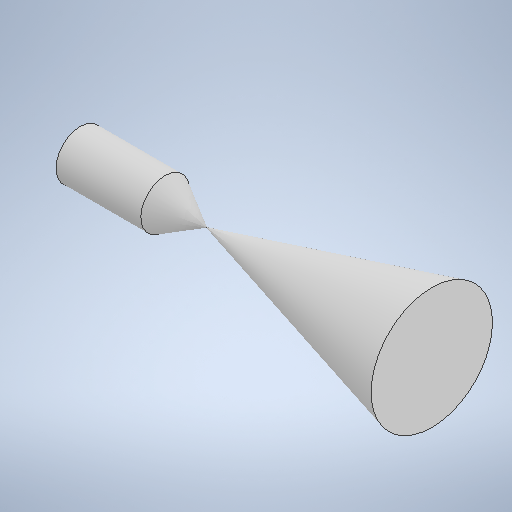
# Autodesk Inventor part: NozzlePath
Saved by Autodesk Inventor 2025.2 (Build 292293000, 293)
## iProperties
Created: 2026-05-12
Part Number: NozzlePath
Material: Generic
Document SubType Name: Modeling
Designer: Simon
Density: 1 g/cm^3
Appearance: Default
Author: Simon
Autodesk Inventor part; units mm, degrees
ref_plane "YZ Plane" through (0, 0, 0) normal (1, 0, 0) x (0, 1, 0)
ref_plane "XZ Plane" through (0, 0, 0) normal (0, 1, 0) x (-1, 0, 0)
ref_plane "XY Plane" through (0, 0, 0) normal (0, 0, 1) x (1, 0, 0)
sketch "Sketch1" plane through (0, 0, 0) normal (0, 0, 1) x (1, 0, 0)
  line L0 (0, -0.0234) -> (0, 1.9766)
  line L1 (0, 1.9766) -> (50, 1.9766)
  line L2 (0, -0.0234) -> (0, 0)
  line L3 (0, 0) -> (50, 0)
  line L4 (0, -0.0234) -> (0, 4.9766)
  line L5 (0, 4.9766) -> (50, 4.9766)
  line L6 (0, -0.0234) -> (0, 3.9766)
  line L7 (0, 3.9766) -> (4, 3.9766)
  line L8 (4, 3.9766) -> (4, 1.9766)
  line L9 (4, 1.9766) -> (4, 9.9766)
  line L10 (4, 1.9766) -> (6.7109, 1.9766) construction
  line L11 (4, 9.9766) -> (7, 9.9766)
  line L12 (7, 9.9766) -> (7, 1.9766)
  line L13 (7, 1.9766) -> (10.4235, 0)
  line L14 (7, 1.9766) -> (9.25, 1.9766) construction
  line L15 (10.4235, 0) -> (28.9964, 4.9766)
  line L16 (10.4235, 0) -> (29.6515, 0) construction
  line L17 (28.9964, 4.9766) -> (28.9964, 6.9766)
  line L18 (28.9964, 6.9766) -> (7, 9.9766)
  line L19 (0, -0.0234) -> (50, -0.0234)
  line L20 (-10, -0.0234) -> (60, -0.0234)
  line L21 (28.9964, 4.9766) -> (28.9964, -0.0234)
  point P0 (28.9964, -0.0234)
  dimension "d0" = 2
  dimension "d1" = 50
  dimension "d2" = 0.0234
  dimension "d3" = 5
  dimension "d4" = 4
  dimension "d5" = 4
  dimension "d6" = 8
  dimension "d7" = 3
  dimension "d8" = 30
  dimension "d9" = 15
  dimension "d10" = 50
  constraints: 44 end point, 8 perpendicular, 8 point on line, 5 horizontal, 2 vertical, 1 equal length
  measures "d0" distance of L0.start L0.end
  measures "d1" distance of L0.end L1.end
  measures "d2" distance of L0.start L2.end
  measures "d3" distance of L0.start L4.end
  measures "d4" distance of L0.start L6.end
  measures "d5" distance of L6.end L8.start
  measures "d6" distance of L8.end L9.end
  measures "d7" distance of L9.end L12.start
  measures "d8" angle of L13 L14
  measures "d9" angle of L16 L15
  measures "d10" distance of L0.start L19.end
revolve "Revolution1" add sketch "Sketch1" angle 360 about axis through (0, -0.0234, 0) along (1, 0, 0) contours L0 L3 L21 L19 | L0 L1 L13 L3 | L15 L1 L21 L3 | L15 L21 L1
body "Solid1"
